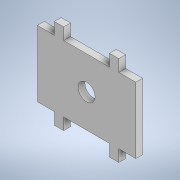
# Autodesk Inventor part: Крепеж колеса
Saved by Autodesk Inventor 2022 (Build 260153000, 153)
## iProperties
Created: 2022-07-10
Part Number: Крепеж колеса
Material: Типовые
Document SubType Name: Modeling
Designer: Константин
Density: 1 g/cm^3
Appearance: По умолчанию
Author: Константин
Autodesk Inventor part; units mm, degrees
ref_plane "YZ Plane" through (0, 0, 0) normal (1, 0, 0) x (0, 1, 0)
ref_plane "XZ Plane" through (0, 0, 0) normal (0, 1, 0) x (-1, 0, 0)
ref_plane "XY Plane" through (0, 0, 0) normal (0, 0, 1) x (1, 0, 0)
sketch "Эскиз1" plane through (0, 0, 0) normal (0, 0, 1) x (1, 0, 0)
  line L0 (14.5, 9.75) -> (14.5, -9.75)
  line L1 (-14.5, -9.75) -> (-14.5, 9.75)
  line L2 (9.5, 9.75) -> (9.5, 13.25)
  line L3 (9.5, 13.25) -> (6.75, 13.25)
  line L4 (6.75, 13.25) -> (6.75, 9.75)
  line L5 (-9.5, 9.75) -> (-9.5, 13.25)
  line L6 (-9.5, 13.25) -> (-6.75, 13.25)
  line L7 (-6.75, 13.25) -> (-6.75, 9.75)
  line L8 (9.5, -9.75) -> (9.5, -13.25)
  line L9 (9.5, -13.25) -> (6.75, -13.25)
  line L10 (6.75, -13.25) -> (6.75, -9.75)
  line L11 (-6.75, -13.25) -> (-6.75, -9.75)
  line L12 (-9.5, -13.25) -> (-6.75, -13.25)
  line L13 (-9.5, -9.75) -> (-9.5, -13.25)
  line L14 (14.5, 9.75) -> (9.5, 9.75)
  line L15 (6.75, 9.75) -> (-6.75, 9.75)
  line L16 (-9.5, 9.75) -> (-14.5, 9.75)
  line L17 (-9.5, -9.75) -> (-14.5, -9.75)
  line L18 (14.5, -9.75) -> (9.5, -9.75)
  line L19 (6.75, -9.75) -> (-6.75, -9.75)
  circle A0 centre (0, 0) radius 2.5
  point P0 (-14.5, 0)
  dimension "d0" = 29
  dimension "d1" = 19.5
  dimension "d2" = 5
  dimension "d3" = 3.5
  dimension "d4" = 2.75
  dimension "d7" = 5
  constraints: 40 end point, 7 perpendicular, 3 horizontal, 2 midpoint, 1 centre point, 1 coincident, 1 horizontal alignment
  measures "d0" distance of L1.end L0.start
  measures "d1" distance of L0.start L0.end
  measures "d2" distance of L0.start L2.start
  measures "d3" distance of L2.start L2.end
  measures "d4" distance of L2.end L3.end
  measures "d7" diameter of A0
extrude "Выдавливание1" add sketch "Эскиз1" along normal blind 2
